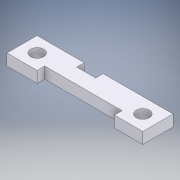
# Autodesk Inventor part: solar_board_holder
Saved by Autodesk Inventor 2018 (Build 220112000, 112)
## iProperties
Created: 2019-04-03
Part Number: solar_board_holder
Material: Generic
Document SubType Name: Modeling
Designer: ZEUSLAP
Density: 1 g/cm^3
Appearance: Default
Mass: 0.656273 g
Surface Area: 7.91489 cm^2
Volume: 0.656273 cm^3
Author: ZEUSLAP
## iProperties of the stored document solar_board_holder_3DPrint.ipt
Created: 2019-04-13
Part Number: solar_board_holder_3DPrint
Material: Generic
Document SubType Name: Modeling
Designer: ZEUSLAP
Density: 1 g/cm^3
Appearance: Default
Author: ZEUSLAP
Autodesk Inventor part; units mm, degrees
ref_plane "YZ Plane" through (0, 0, 0) normal (1, 0, 0) x (0, 1, 0)
ref_plane "XZ Plane" through (0, 0, 0) normal (0, 1, 0) x (-1, 0, 0)
ref_plane "XY Plane" through (0, 0, 0) normal (0, 0, 1) x (1, 0, 0)
sketch "Sketch" plane through (0, 0, 0) normal (0, 0, 1) x (1, 0, 0)
  line L0 (-18, -4) -> (-18, 4)
  circle A0 centre (-14, 0) radius 1.75
  circle A1 centre (14, 0) radius 1.75
  line L1 (-10, -2) -> (-10, -4)
  line L2 (10.5, -2) -> (10.5, -4)
  line L3 (-18, -4) -> (-10, -4)
  line L4 (10.5, -4) -> (18, -4)
  line L5 (-5.5, 4) -> (-5.5, 2)
  line L6 (-5.5, 2) -> (-0.5, 2)
  line L7 (-0.5, 2) -> (-0.5, 4)
  line L8 (-0.5, 4) -> (5.8141, 4)
  line L9 (-0.5, 4) -> (18, 4)
  line L10 (18, 4) -> (18, -4)
  line L11 (-10, -2) -> (10.5, -2)
  line L12 (-5.5, 4) -> (-18, 4)
  line L13 (0, 15.191) -> (0, -14.809) construction
  point P0 (0, 0)
  point P1 (18, 0)
  dimension "d18" = 3.5
  dimension "d34" = 5
  dimension "d35" = 20.5
  dimension "d36" = 2
  dimension "d39" = 36
  dimension "d41" = 8
  dimension "d45" = 12.5
  dimension "d48" = 8
  dimension "d49" = 14
  constraints: 28 end point, 6 perpendicular, 4 parallel, 3 horizontal, 2 centre point, 2 vertical, 1 equal radius, 1 horizontal alignment, 1 midpoint, 1 point on line, 2 other
  measures "d18" diameter of A0
  measures "d34" distance between parallel lines of L7 L5
  measures "d35" distance between parallel lines of L2 L1
  measures "d36" distance of L1.start L1.end
  measures "d39" distance between parallel lines of L10 L0
  measures "d41" distance of L0.start L0.end
  measures "d45" distance of L5.start L0.end
  measures "d48" distance of L0.start L1.end
  measures "d49" distance of point (0, 0) A0.centre
extrude "Extrusion" add sketch "Sketch" along normal blind 3
body "Solid4"
